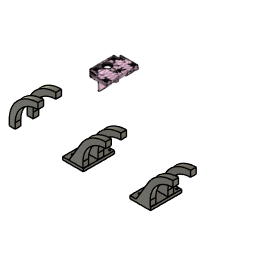
Robotics Gripper v5 (Autodesk Fusion 360 design; units mm, degrees)
Autodesk Fusion 360 part; units mm, degrees
note: some values were not read from the file. Chosen so that the rebuilt part matches the saved one: which bodies a step acts on; that a step has no effect. Set by a fixed rule: the direction of a hole.
form "Form1" [no effect]
other "Base Mesh Feature1"
other "Modify1"
sketch "Sketch1" plane through (0, 0, 0) normal (0, 0, 1) x (1, 0, 0)
  line L0 (0, 0) -> (36.75, 0)
  line L1 (36.75, 0) -> (36.75, 57.51)
  line L2 (36.75, 57.51) -> (0, 57.51)
  line L3 (0, 57.51) -> (0, 0)
  dimension "d1" = 36.75
  dimension "d2" = 57.51
  constraint coincident L0.start L3.end
  constraint horizontal L0
  constraint perpendicular L0 L1
  constraint perpendicular L1 L2
  constraint perpendicular L0 L3
  measures "d1" distance of L0.start L0.end
  measures "d2" distance of L0.end L1.end
extrude "Extrude1" add sketch "Sketch1" along normal blind 5 makes body 1
other "Modify2"
other "Modify3"
other "Modify4"
sketch "Sketch2" plane through (0, 0, 0) normal (0, -1, 0) x (1, 0, 0)
  line L0 (0, 0) -> (36.75, 0)
  line L1 (36.75, 0) -> (36.75, 5)
  line L2 (36.75, 5) -> (0, 5)
  line L3 (0, 5) -> (0, 0)
  arc A0 (35, 40) -> (0, 5) centre (35, 5) ccw
  arc A1 (35, 30) -> (10, 5) centre (35, 5) ccw
  line L4 (35, 40) -> (35, 30)
  line L5 (0, 5) -> (10, 5)
  constraint coincident L2.end L3.start
  constraint tangent L3 A0
  constraint coincident L2 A1.end
  constraint coincident A0.centre A1.centre
  constraint vertical L4
extrude "Extrude2" add sketch "Sketch2" against normal blind 13.8775 contours L2 A0 A1 L4 L5 bodies 1
copy_body "Body->Comp1" bodies 1 removing the originals makes body 2 in component "Component"
other "Body->Comp1'"
split "Split1" by plane through (0, 0, 5) normal (0, 0, 1) bodies 2 makes body 3 at (0.0396, 9.2517, 6.6654) in component "Component"
other "Modify1'" in component "OpenManipulator_Finger_Adapter_V6"
other "Modify2'" in component "OpenManipulator_Finger_Adapter_V6"
delete_body "RemoveBody1" bodies 3 in component "Component"
sketch "Sketch3" plane through (0, 0, 0) normal (0, 1, 0) x (1, 0, 0)
  circle A0 centre (65.5241, -27.502) radius 27.5
  arc A1 (25.1427, -15.1295) -> (65.6668, -55.6483) centre (65.6668, -15.1242) ccw
  line L0 (25.1427, -15.1295) -> (25.1427, -5)
  line L1 (65.6668, -55.6483) -> (65.6668, -66.1995)
  arc A2 (14.5914, -15.1242) -> (65.6668, -66.1995) centre (65.6668, -15.1242) ccw
  line L2 (14.5914, -15.1242) -> (14.5914, -5)
  line L3 (14.5914, -5) -> (25.1427, -5)
  line L4 (0, -5) -> (21.8853, -41.4276)
  line L5 (0, -5) -> (14.5914, -5)
  dimension "d7" = 55
  constraint vertical L0
  constraint vertical L1
  constraint coincident A1.centre A2.centre
  constraint tangent A2 L2
  constraint vertical L2
  constraint perpendicular L0 L3
  constraint coincident A2 L4.end
  constraint tangent A2 L4
  constraint perpendicular L2 L5
  measures "d7" diameter of A0
extrude "Extrude1'" add sketch "Sketch3" along normal blind 10 contours A1 L0 L1 A2 L2 L3 bodies 2 in component "Component"
split "Split2" by plane through (0, 0, 5) normal (0, 0, 1) bodies 2 makes body 4 at (21.6256, 10, 11.7512) in component "Component"
copy_body "CopyPasteBodies1" bodies 4 makes body 5 in component "Component"
move_body "Move1" bodies 4 to x (1, 0, 0) y (0, 1, 0) z (0, 0, 1) at (0, 32, 0) in component "Component"
combine "Combine1" operation add target body 2 tool bodies 5 4 in component "Component"
move_body "Move2" bodies 2 to x (1, 0, 0) y (0, 1, 0) z (0, 0, 1) at (-80, 0, 0) in component "Component"
sketch "BAse" plane through (0, 0, 0) normal (0, 0, 1) x (1, 0, 0)
  line L0 (0, 0) -> (36.75, 0)
  line L1 (36.75, 0) -> (36.75, 55.51)
  line L2 (36.75, 55.51) -> (0, 55.51)
  line L3 (0, 55.51) -> (0, 0)
  point P0 (5.25, 11.755)
  point P1 (5.25, 43.755)
  point P2 (31.75, 3.755)
  point P3 (31.75, 51.755)
  dimension "d10" = 36.75
  dimension "d11" = 55.51
  constraint horizontal L0
  constraint vertical L1
  constraint horizontal L2
  constraint vertical L3
  constraint coincident L0.start L3.end
  measures "d10" distance of L0.start L0.end
  measures "d11" distance of L0.start L2.end
extrude "Extrude3" add sketch "BAse" along normal blind 5 separate body makes body 6
hole "Hole1" at (31.75, 3.755, 0) direction (0, 0, 1) diameter 3 depth 25 tip angle 118 bodies 6
hole "Hole2" at (5.25, 11.755, 0) direction (0, 0, 1) diameter 3 depth 25 tip angle 118 bodies 6
hole "Hole3" at (5.25, 43.755, 0) direction (0, 0, 1) diameter 3 depth 25 tip angle 118 bodies 6
hole "Hole4" at (31.75, 51.755, 0) direction (0, 0, 1) diameter 3 depth 25 tip angle 118 bodies 6
move_body "Move3" bodies 2 to x (1, 0, 0) y (0, 1, 0) z (0, 0, 1) at (80, 0, 0) in component "Component"
split "Split3" by plane through (0, 0, 5) normal (0, 0, 1) bodies 2 makes body 7 at (21.6256, 10, 11.7512) makes body 8 at (21.6256, 42, 11.7512) in component "Component"
move_body "Move4" bodies 2 to x (1, 0, 0) y (0, 1, 0) z (0, 0, 1) at (-73.3417, 46.2114, 0) in component "Component"
delete_body "RemoveBody2" bodies 2 in component "Component"
copy_body "CutPasteBodies3" bodies 7 8 removing the originals makes body 9 makes body 10
move_body "Move3'" bodies 10 9 to x (1, 0, 0) y (0, 1, 0) z (0, 0, 1) at (90, 0, 0)
extrude "Extrude2'" add sketch "Sketch3" along normal blind 10 contours A1 L0 L1 A2 L2 L3 | A2 L2 L4 L5 makes body 11 in component "Component"
copy_body "CopyPasteBodies2" bodies 11 makes body 12 in component "Component"
move_body "Move5" bodies 12 to x (1, 0, 0) y (0, 1, 0) z (0, 0, 1) at (0, 27, 0) in component "Component"
move_body "Move6" bodies 11 12 to x (1, 0, 0) y (0, 1, 0) z (0, 0, 1) at (11, 0, 0) in component "Component"
copy_body "CutPasteBodies3'" bodies 6 removing the originals makes body 13 in component "Component"
move_body "Move7" bodies 11 12 13 to x (1, 0, 0) y (0, 1, 0) z (0, 0, 1) at (-120, 0, 0) in component "Component"
copy_body "CopyPasteBodies1'" bodies 11 13 12 makes body 14 makes body 15 makes body 16 in component "Gripper"
move_body "Move1'" bodies 14 15 16 to x (1, 0, 0) y (0, 1, 0) z (0, 0, 1) at (120, 0, 0) in component "Gripper"
move_body "Move4'" bodies 9 10 to x (1, 0, 0) y (0, 1, 0) z (0, 0, 1) at (-320, 0, 0)
delete_body "RemoveBody1'" bodies 16 in component "Gripper"
copy_body "CopyPasteBodies3" bodies 14 makes body 17 in component "Gripper"
move_body "Move3''" bodies 17 to x (1, 0, 0) y (0, 1, 0) z (0, 0, 1) at (0, 31.6325, 0) in component "Gripper"
combine "Combine1'" operation add target body 14 tool bodies 15 17 in component "Gripper"
component "OpenManipulator_Finger_Adapter_V6" placed x (1, 0, 0) y (0, -1, 0) z (0, 0, -1) at (-173.2548, 277.5224, 147.2891)
component "Component" placed x (1, 0, 0) y (0, 1, 0) z (0, 0, 1) at (0, 0, 0)
component "Gripper" placed x (1, 0, 0) y (0, 1, 0) z (0, 0, 1) at (0, 0, 0)
component "Gripper" placed x (1, 0, 0) y (0, 1, 0) z (0, 0, 1) at (0, 0, 0)
